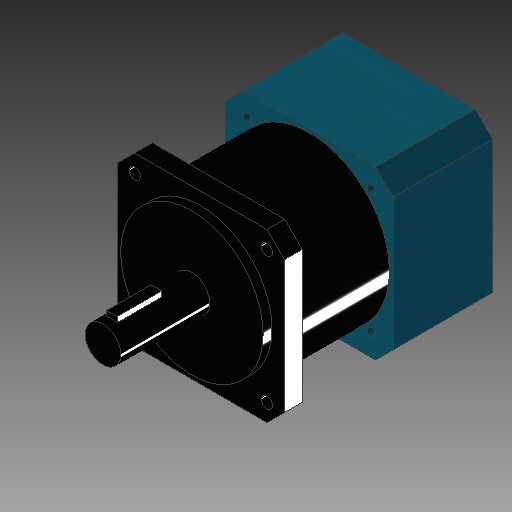
# Autodesk Inventor part: 2312_Gear Box_V1
Saved by Autodesk Inventor 2020 (Build 240168000, 168)
## iProperties
Created: 2019-09-12
Part Number: 2312_Gear Box_V1
Material: Generic
Document SubType Name: Modeling
Designer: MPI
Density: 1 g/cm^3
Appearance: Default
Mass: 925.453 g
Surface Area: 696.504 cm^2
Volume: 925.453 cm^3
Author: MPI
Autodesk Inventor part; units mm, degrees
ref_plane "YZ Plane" through (0, 0, 0) normal (1, 0, 0) x (0, 1, 0)
ref_plane "XZ Plane" through (0, 0, 0) normal (0, 1, 0) x (-1, 0, 0)
sketch "Sketch1" plane through (0, 0, 0) normal (0, 0, 1) x (1, 0, 0)
  line L0 (-37.2, 47) -> (37.2, 47)
  line L1 (47, 37.2) -> (47, -37.2)
  line L2 (37.2, -47) -> (-37.2, -47)
  line L3 (-47, -37.2) -> (-47, 37.2)
  circle A0 centre (0, 0) radius 52.5 construction
  line L4 (-37.125, 58) -> (-37.125, -64) construction
  line L5 (37.125, 58) -> (37.125, -64) construction
  line L6 (-69, 37.125) -> (85, 37.125) construction
  line L7 (-58, -37.125) -> (77, -37.125) construction
  circle A1 centre (-37.125, 37.125) radius 3.175
  circle A2 centre (37.125, 37.125) radius 3.175
  circle A3 centre (37.125, -37.125) radius 3.175
  circle A4 centre (-37.125, -37.125) radius 3.175
  line L8 (-37.2, 47) -> (-47, 37.2)
  line L9 (37.2, 47) -> (47, 37.2)
  line L10 (-47, -37.2) -> (-37.2, -47)
  line L11 (37.2, -47) -> (47, -37.2)
  point P0 (-47, 47)
  point P1 (47, -47)
  point P2 (47, 47)
  point P3 (-47, -47)
  dimension "d0" = 94
  dimension "d1" = 47
  dimension "d2" = 47
  dimension "d3" = 105
  dimension "d4" = 74.25
  dimension "d5" = 37.125
  dimension "d6" = 74.25
  dimension "d7" = 37.125
  dimension "d8" = 6.35
  dimension "d9" = 6.35
  dimension "d10" = 6.35
  dimension "d11" = 6.35
  dimension "d12" = 9.8
  dimension "d13" = 9.8
  dimension "d14" = 9.8
  dimension "d15" = 9.8
  dimension "d16" = 9.8
  dimension "d17" = 9.8
  dimension "d18" = 9.8
  dimension "d19" = 9.8
  constraints: 24 end point, 10 point on line, 5 centre point, 3 horizontal, 2 parallel, 2 perpendicular, 2 vertical, 1 coincident
  measures "d0" distance of point (-47, 47) point (47, 47)
  measures "d1" horizontal distance of point (0, 0) point (-47, 47)
  measures "d2" horizontal distance of point (0, 0) point (47, 47)
  measures "d3" diameter of A0
  measures "d4" distance between parallel lines of L5 L4
  measures "d5" distance from line of point (0, 0) L4
  measures "d6" distance from line of L7.start L6
  measures "d7" distance from line of L7 point (0, 0)
  measures "d8" diameter of A1
  measures "d9" diameter of A2
  measures "d10" diameter of A3
  measures "d11" diameter of A4
  measures "d12" distance of L0.start point (-47, 47)
  measures "d13" distance of L3.end point (-47, 47)
  measures "d14" distance of L0.end point (47, 47)
  measures "d15" distance of L1.start point (47, 47)
  measures "d16" distance of L3.start point (-47, -47)
  measures "d17" distance of L2.end point (-47, -47)
  measures "d18" distance of L2.start point (47, -47)
  measures "d19" distance of L1.end point (47, -47)
extrude "Extrusion1" add sketch "Sketch1" along normal blind 10
sketch "Sketch2" plane through (0, 0, 10) normal (0, 0, 1) x (1, 0, 0)
  circle A0 centre (0, 0) radius 40
  dimension "d22" = 80
  constraints: 1 centre point, 1 coincident
  measures "d22" diameter of A0
extrude "Extrusion2" add sketch "Sketch2" along normal blind 5
sketch "Sketch3" plane through (0, 0, 15) normal (0, 0, 1) x (1, 0, 0)
  circle A0 centre (0, 0) radius 10
  dimension "d25" = 20
  constraints: 1 centre point, 1 coincident
  measures "d25" diameter of A0
extrude "Extrusion3" add sketch "Sketch3" along normal blind 50
ref_plane "Work Plane1" through (0, 0, 60) normal (0, 0, 1) x (1, 0, 0)
sketch "Sketch5" plane through (0, 0, 60) normal (0, 0, 1) x (1, 0, 0)
  line L0 (-3, 12.5) -> (3, 12.5)
  line L1 (3, 12.5) -> (3, 7.2)
  line L2 (3, 7.2) -> (-3, 7.2)
  line L3 (-3, 7.2) -> (-3, 12.5)
  point P0 (0, 0)
  dimension "d29" = 6
  dimension "d30" = 3
  dimension "d31" = 12.5
  constraints: 8 end point, 2 parallel, 1 horizontal, 1 perpendicular
  measures "d29" distance of L0.start L0.end
  measures "d30" distance from line of point (0, 0) L3
  measures "d31" distance from line of point (0, 0) L0
extrude "Extrusion4" add sketch "Sketch5" against normal blind 25
sketch "Sketch6" plane through (0, 0, 0) normal (0, 0, -1) x (-1, 0, 0)
  circle A0 centre (0, 0) radius 45
  dimension "d34" = 90
  constraints: 1 centre point, 1 coincident
  measures "d34" diameter of A0
extrude "Extrusion5" add sketch "Sketch6" along normal blind 51
sketch "Sketch8" plane through (0, 0, -51) normal (0, 0, -1) x (-1, 0, 0)
  line L0 (-37.2, 47) -> (37.2, 47)
  line L1 (47, 37.2) -> (47, -37.2)
  line L2 (37.2, -47) -> (-37.2, -47)
  line L3 (-47, -37.2) -> (-47, 37.2)
  line L4 (-37.2, 47) -> (37.2, 47) projected
  line L5 (47, 37.2) -> (47, -37.2) projected
  line L6 (37.2, -47) -> (-37.2, -47) projected
  line L7 (-47, -37.2) -> (-47, 37.2) projected
  circle A0 centre (-34.798, 34.798) radius 2.5
  circle A1 centre (34.798, 34.798) radius 2.5
  circle A2 centre (34.798, -34.798) radius 2.5
  circle A3 centre (-34.798, -34.798) radius 2.5
  line L8 (-37.2, 47) -> (-47, 37.2)
  line L9 (37.2, 47) -> (47, 37.2)
  line L10 (47, -37.2) -> (37.2, -47)
  line L11 (-37.2, -47) -> (-47, -37.2)
  point P0 (0, 0)
  point P1 (-47, 47)
  point P2 (47, -47)
  point P3 (47, 47)
  point P4 (-47, -47)
  dimension "d38" = 5
  dimension "d39" = 5
  dimension "d40" = 5
  dimension "d41" = 5
  dimension "d42" = 69.596
  dimension "d43" = 69.596
  dimension "d44" = 69.596
  dimension "d45" = 69.596
  dimension "d46" = 34.798
  dimension "d47" = 34.798
  dimension "d48" = 34.798
  dimension "d49" = 34.798
  dimension "d50" = 9.8
  dimension "d51" = 9.8
  dimension "d52" = 9.8
  dimension "d53" = 9.8
  dimension "d54" = 9.8
  dimension "d55" = 9.8
  dimension "d56" = 9.8
  dimension "d57" = 9.8
  constraints: 16 end point, 8 point on line, 4 centre point, 4 collinear, 2 parallel, 1 horizontal, 1 perpendicular
  measures "d38" diameter of A0
  measures "d39" diameter of A1
  measures "d40" diameter of A2
  measures "d41" diameter of A3
  measures "d42" distance of A1.centre A0.centre
  measures "d43" distance of A2.centre A1.centre
  measures "d44" distance of A2.centre A3.centre
  measures "d45" distance of A3.centre A0.centre
  measures "d46" horizontal distance of point (0, 0) A0.centre
  measures "d47" horizontal distance of point (0, 0) A1.centre
  measures "d48" horizontal distance of A0.centre point (0, 0)
  measures "d49" horizontal distance of point (0, 0) A3.centre
  measures "d50" distance of L0.start point (-47, 47)
  measures "d51" distance of L3.end point (-47, 47)
  measures "d52" distance of L0.end point (47, 47)
  measures "d53" distance of L1.start point (47, 47)
  measures "d54" distance of L1.end point (47, -47)
  measures "d55" distance of L2.start point (47, -47)
  measures "d56" distance of L2.end point (-47, -47)
  measures "d57" distance of L3.start point (-47, -47)
extrude "Extrusion6" add sketch "Sketch8" along normal blind 56
sketch "Sketch9" plane through (0, 0, -107) normal (0, 0, -1) x (-1, 0, 0)
  circle A0 centre (0, 0) radius 6.35
  dimension "d60" = 12.7
  constraints: 1 centre point, 1 coincident
  measures "d60" diameter of A0
extrude "Extrusion7" cut sketch "Sketch9" against normal blind 40
equation "\"d13\" = d12"
equation "\"d14\" = d12"
equation "\"d15\" = d14"
equation "\"d16\" = d12"
equation "\"d17\" = d16"
equation "\"d18\" = d12"
equation "\"d19\" = d18"
equation "\"d51\" = d50"
equation "\"d52\" = d50"
equation "\"d53\" = d52"
equation "\"d54\" = d50"
equation "\"d55\" = d54"
equation "\"d56\" = d50"
equation "\"d57\" = d56"
body "Solid1"
